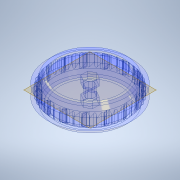
# Autodesk Inventor part: ratchet
Saved by Autodesk Inventor 2022 (Build 260153000, 153)
## iProperties
Created: 2021-10-28
Part Number: ratchet
Material: Generic
Document SubType Name: Modeling
Designer: Chris Spooner
Density: 1 g/cm^3
Appearance: Clear - Blue
Author: Chris Spooner
Autodesk Inventor part; units mm, degrees
ref_plane "YZ Plane" through (0, 0, 0) normal (1, 0, 0) x (0, 1, 0)
ref_plane "XZ Plane" through (0, 0, 0) normal (0, 1, 0) x (-1, 0, 0)
ref_plane "XY Plane" through (0, 0, 0) normal (0, 0, 1) x (1, 0, 0)
sketch "Sketch1" plane through (0, 0, 0) normal (0, 0, 1) x (1, 0, 0)
  line L0 (22.86, 6.35) -> (0, 6.35)
  line L1 (0, 6.35) -> (0, -6.35)
  line L2 (0, -6.35) -> (22.86, -6.35)
  line L3 (22.86, -6.35) -> (22.86, 6.35)
  line L4 (22.86, 6.35) -> (0, -6.35) construction
  line L5 (0, 6.35) -> (22.86, -6.35) construction
  line L6 (16.3859, 6.35) -> (19.05, 3.175)
  line L7 (19.05, 3.175) -> (19.05, -3.175)
  line L8 (19.05, -3.175) -> (16.3859, -6.35)
  line L9 (17.7122, 6.35) -> (21.59, 1.7286)
  line L10 (21.59, 1.7286) -> (21.59, -1.7286)
  line L11 (21.59, -1.7286) -> (17.7122, -6.35)
  point P0 (0, 0)
  point P1 (11.43, 0)
  point P2 (11.43, 0)
  point P3 (0, 0)
  point P4 (19.05, 0)
  point P5 (11.43, 0)
  point P6 (21.59, 0)
  dimension "d0" = 12.7
  dimension "d1" = 22.86
  dimension "d2" = 50
  dimension "d3" = 19.05
  dimension "d4" = 6.35
  dimension "d5" = 2.54
  dimension "d6" = 1.016
  constraints: 24 end point, 7 midpoint, 4 horizontal alignment, 4 parallel, 4 point on line, 2 vertical, 1 coincident, 1 equal length, 1 horizontal, 1 perpendicular
  measures "d0" distance of L0.end L1.end
  measures "d1" distance of L0.start L0.end
  measures "d2" angle of L0 L6
  measures "d3" distance between parallel lines of L1 L7
  measures "d4" distance of L6.end L7.end
  measures "d5" distance between parallel lines of L7 L10
  measures "d6" distance between parallel lines of L6 L9
revolve "Revolution1" add sketch "Sketch1" angle 360 about axis through (0, 6.35, 0) along (0, -1, 0) contours L3 L2 L11 L10 L9 L0 | L6 L7 L8 L2 L1 L0
sketch "Sketch2" plane through (0, 0, 0) normal (0, 1, 0) x (-1, 0, 0)
  circle A0 centre (0, 0) radius 21.59 projected
  line L0 (0, -21.59) -> (0, -19.685)
  line L1 (0, -19.685) -> (-2.9491, -21.3876)
  arc A1 (-2.9491, -21.3876) -> (0, -21.59) centre (0, 0) ccw
  dimension "d8" = 1.905
  dimension "d9" = 60
  constraints: 4 end point, 4 point on circle, 1 centre point, 1 concentric, 1 vertical, 1 vertical alignment
  measures "d8" distance of L0.start L0.end
  measures "d9" angle of L0 L1
extrude "Extrusion1" add sketch "Sketch2" against normal up to surface (12.7 mm away) from surface at 6.35 contours L1 L0 A0 picked at (-1.6395, -20.8575)
fillet "Fillet2" radius 0.635 1 edges at (0, 0, -19.685)
pattern_circular "Circular Pattern1" count 45 over 360 about axis through (0, 0, 0) along (0, -1, 0) of "Extrusion1", "Fillet2"
sketch "Sketch3" plane through (0, 0, 0) normal (0, 1, 0) x (-1, 0, 0)
  circle A0 centre (0, 0) radius 22.86 projected
  circle A1 centre (0, 0) radius 17.7122 projected
  line L0 (0, -20.7849) -> (0, -21.59) projected
  line L1 (0, -21.59) -> (0, -20.7849) projected
  circle A2 centre (0, 0) radius 19.05 projected
  line L2 (2.9026, -18.8276) -> (0.381, -20.4651)
  line L3 (0.381, -20.4651) -> (0.381, -19.8594)
  line L4 (0.381, -19.8594) -> (1.7517, -18.9693)
  line L5 (0.0562, -21.5899) -> (1.8729, -20.1706) projected
  point P0 (2.3929, -19.7643)
  dimension "d15" = 0.508
  dimension "d16" = 5
  dimension "d17" = 0.381
  dimension "d23" = 0.508
  constraints: 6 end point, 2 parallel, 2 point on circle
  measures "d15" distance between parallel lines of L4 L2
  measures "d16" angle of L5 L2
  measures "d17" distance between parallel lines of L0 L3
  measures "d23" distance from line of L2 point (2.393, -19.764)
extrude "Extrusion2" add sketch "Sketch3" along normal mid plane 6.35 contours A2 L2 L3 L4
fillet "Fillet1" radius 0.0635 1 edges at (-1.7517, 0, -18.9693)
pattern_circular "Circular Pattern2" count 15 over 360 about axis through (0, 0, 0) along (0, -1, 0) of "Extrusion2", "Fillet1"
chamfer "Chamfer1" distance 3.175 angle 45 2 edges at (-22.86, 6.35, 0) (-22.86, -6.35, 0)
ref_plane "Work Plane1" through (0, 0, 0) normal (0, 1, 0) x (1, 0, 0)
sketch "Sketch5" plane through (0, 0, 0) normal (0, 1, 0) x (1, 0, 0)
  line L0 (0, -3.6662) -> (-3.175, -1.8331)
  line L1 (-3.175, -1.8331) -> (-3.175, 1.8331)
  line L2 (-3.175, 1.8331) -> (0, 3.6662)
  line L3 (0, 3.6662) -> (3.175, 1.8331)
  line L4 (3.175, 1.8331) -> (3.175, -1.8331)
  line L5 (3.175, -1.8331) -> (0, -3.6662)
  line L6 (0, -3.0796) -> (-2.667, -1.5398)
  line L7 (-2.667, -1.5398) -> (-2.667, 1.5398)
  line L8 (-2.667, 1.5398) -> (0, 3.0796)
  line L9 (0, 3.0796) -> (2.667, 1.5398)
  line L10 (2.667, 1.5398) -> (2.667, -1.5398)
  line L11 (2.667, -1.5398) -> (0, -3.0796)
  line L12 (0, -2.493) -> (-2.159, -1.2465)
  line L13 (-2.159, -1.2465) -> (-2.159, 1.2465)
  line L14 (-2.159, 1.2465) -> (0, 2.493)
  line L15 (0, 2.493) -> (2.159, 1.2465)
  line L16 (2.159, 1.2465) -> (2.159, -1.2465)
  line L17 (2.159, -1.2465) -> (0, -2.493)
  point P0 (0, 0)
  point P1 (0, 0)
  point P2 (0, 0)
  point P3 (0, 0)
  dimension "d39" = 6.35
  dimension "d40" = 0.508
  dimension "d41" = 0.508
  constraints: 36 end point, 3 coincident, 1 vertical, 39 other
  measures "d39" distance between parallel lines of L1 L4
  measures "d40" distance between parallel lines of L6 L0
  measures "d41" distance between parallel lines of L12 L6
extrude "Extrusion6" cut sketch "Sketch5" along normal through all both and the other way through all contours L0 L1 L2 L3 L4 L5 | L6 L7 L8 L9 L10 L11 | L12 L13 L14 L15 L16 L17
extrude "Extrusion10" add sketch "Sketch5" along normal mid plane 5.08 contours L0 L1 L2 L3 L4 L5 | L6 L7 L8 L9 L10 L11 | L12 L13 L14 L15 L16 L17
extrude "Extrusion11" cut sketch "Sketch5" along normal through all both and the other way through all contours L12 L13 L14 L15 L16 L17
body "Solid1"
